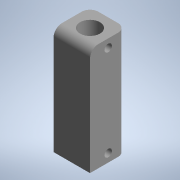
# Autodesk Inventor part: microscope_mount
Saved by Autodesk Inventor 2022 (Build 260153000, 153)
## iProperties
Part Number: microscope_mount
Material: Allgemein
Document SubType Name: Modellieren
Designer: Niclas
Appearance: Vorgabe
Author: Niclas
Autodesk Inventor part; units mm, degrees
ref_plane "YZ-Ebene" through (0, 0, 0) normal (1, 0, 0) x (0, 1, 0)
ref_plane "XZ-Ebene" through (0, 0, 0) normal (0, 1, 0) x (-1, 0, 0)
ref_plane "XY-Ebene" through (0, 0, 0) normal (0, 0, 1) x (1, 0, 0)
sketch "Skizze1" plane through (0, 0, 0) normal (0, 1, 0) x (-1, 0, 0)
  line L0 (22, 0) -> (0, 0)
  line L1 (0, 0) -> (0, -17)
  line L2 (5, -22) -> (17, -22)
  line L3 (22, -17) -> (22, 0)
  arc A0 (17, -22) -> (22, -17) centre (17, -17) ccw
  arc A1 (0, -17) -> (5, -22) centre (5, -17) ccw
  point P0 (0, 0)
  point P1 (22, 0)
  point P2 (0, -22)
  point P3 (0, 0)
  point P4 (22, -22)
  point P5 (0, 0)
  point P6 (0, 0)
  point P7 (0, 0)
  point P8 (22, 0)
  point P9 (22, 0)
  point P10 (22, 0)
  point P11 (0, -22)
  point P12 (0, -22)
  point P13 (0, -22)
  point P14 (22, 0)
  dimension "d0" = 22
  dimension "d1" = 22
  dimension "d32" = 5
  dimension "d37" = 5
  constraints: 16 point on line, 10 end point, 5 horizontal, 4 point on circle, 4 tangent, 4 vertical, 3 coincident, 2 centre point, 2 parallel, 1 perpendicular, 16 other
  measures "d0" distance of point (22, -22) point (22, 0)
  measures "d1" distance of point (0, -22) point (22, -22)
  measures "d32" radius of A0
  measures "d37" radius of A1
extrude "Extrusion1" add sketch "Skizze1" along normal blind 65
sketch "Skizze2" plane through (0, 65, 0) normal (0, 1, 0) x (1, 0, 0)
  circle A0 centre (-11, 11) radius 6
  line L0 (-5, 22) -> (-17, 22) projected
  line L1 (0, 0) -> (0, 17) projected
  point P0 (0, 22)
  point P1 (-22, 22)
  point P2 (0, 22)
  dimension "d6" = 12
  dimension "d17" = 11
  dimension "d18" = 11
  constraints: 1 centre point
  measures "d6" diameter of A0
  measures "d17" distance from line of L1 A0.centre
  measures "d18" distance from line of L0 A0.centre
extrude "Extrusion2" cut sketch "Skizze2" against normal blind 84
sketch "Skizze3" plane through (0, 0, 0) normal (1, 0, 0) x (0, 0, -1)
  circle A0 centre (11, 60) radius 2.25
  circle A1 centre (11, 5) radius 2.25
  line L0 (22, 0) -> (22, 65) projected
  line L1 (0, 0) -> (17, 0) projected
  line L2 (0, 0) -> (0, 84) projected
  point P0 (22, 0)
  dimension "d11" = 5
  dimension "d12" = 55
  dimension "d13" = 4.5
  dimension "d14" = 4.5
  dimension "d28" = 11
  dimension "d29" = 11
  constraints: 2 centre point
  measures "d11" distance from line of L1 A1.centre
  measures "d12" distance of A0.centre A1.centre
  measures "d13" diameter of A1
  measures "d14" diameter of A0
  measures "d28" distance from line of L0 A0.centre
  measures "d29" distance from line of L0 A1.centre
extrude "Extrusion3" cut sketch "Skizze3" against normal blind 12
sketch "Skizze6" plane through (-22, 0, -17) normal (-1, 0, 0) x (0, 0, 1)
  line L0 (0, 0) -> (17, 0) projected
  line L1 (0, 65) -> (-5, 65) projected
  line L2 (12, 0) -> (-5, 0)
  line L3 (-5, 0) -> (-5, 65)
  line L4 (-5, 65) -> (12, 65)
  line L5 (17, 60) -> (17, 5)
  arc A0 (17, 60) -> (12, 65) centre (12, 60) ccw
  line L6 (17, 0) -> (-5, 0)
  line L7 (-5, 0) -> (-5, 65)
  line L8 (-5, 65) -> (17, 65)
  line L9 (17, 65) -> (17, 0)
  point P0 (12, 65)
  dimension "d33" = 5
  constraints: 16 end point, 4 parallel, 2 horizontal, 2 perpendicular, 2 point on circle, 2 point on line, 2 tangent, 1 centre point
  measures "d33" radius of A0
extrude "Extrusion5" cut sketch "Skizze6" against normal blind 25 contours A0 L8 L9
